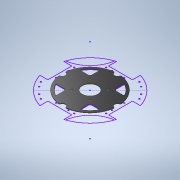
# Autodesk Inventor part: board
Saved by Autodesk Inventor 2020 (Build 240168000, 168)
## iProperties
Created: 2024-09-14
Part Number: board
Material: Типовые
Document SubType Name: Modeling
Designer: Ivan
Density: 1 g/cm^3
Appearance: Глянцевая — черная
Author: Ivan
Autodesk Inventor part; units mm, degrees
ref_plane "YZ Plane" through (0, 0, 0) normal (1, 0, 0) x (0, 1, 0)
ref_plane "XZ Plane" through (0, 0, 0) normal (0, 1, 0) x (-1, 0, 0)
ref_plane "XY Plane" through (0, 0, 0) normal (0, 0, 1) x (1, 0, 0)
sketch "Эскиз1" plane through (0, 0, 0) normal (0, 1, 0) x (-1, 0, 0)
  circle A0 centre (0, 0) radius 72.2724
  line L0 (46.8072, -8) -> (71.8282, -8)
  line L1 (46.8072, 8) -> (71.8282, 8)
  line L2 (-8, 46.8072) -> (-8, 71.8282)
  line L3 (8, 46.8072) -> (8, 71.8282)
  line L4 (-46.8072, -8) -> (-71.8282, -8)
  line L5 (-46.8072, 8) -> (-71.8282, 8)
  line L6 (8, -46.8072) -> (8, -71.8282)
  line L7 (-8, -46.8072) -> (-8, -71.8282)
  circle A1 centre (0, 0) radius 20
  point P0 (0, 0)
  point P1 (71.0292, -13.3471)
  point P2 (71.0292, 13.3471)
  constraints: 16 end point, 2 centre point, 1 horizontal, 1 point on circle
sketch "Эскиз4" plane through (0, 0, 0) normal (0, 1, 0) x (-1, 0, 0)
  line L0 (31, 34.7373) -> (31, 58.0259)
  line L1 (34.72, 31.0173) -> (58.0086, 31.0173)
  arc A0 (34.72, 31.0173) -> (31, 34.7373) centre (0, 0.0173) ccw
  arc A1 (58.0086, 31.0173) -> (31, 58.0259) centre (0, 0.0173) ccw
  line L2 (-58.0173, 31.0259) -> (-34.7286, 31.0259)
  arc A2 (-31.0086, 58.0346) -> (-58.0173, 31.0259) centre (-0.0086, 0.0259) ccw
  line L3 (-31.0086, 34.7459) -> (-31.0086, 58.0346)
  arc A3 (-31.0086, 34.7459) -> (-34.7286, 31.0259) centre (-0.0086, 0.0259) ccw
  line L4 (-31.0173, -57.9914) -> (-31.0173, -34.7027)
  arc A4 (-58.0259, -30.9827) -> (-31.0173, -57.9914) centre (-0.0173, 0.0173) ccw
  line L5 (-34.7373, -30.9827) -> (-58.0259, -30.9827)
  arc A5 (-34.7373, -30.9827) -> (-31.0173, -34.7027) centre (-0.0173, 0.0173) ccw
  line L6 (58, -30.9914) -> (34.7114, -30.9914)
  arc A6 (30.9914, -58) -> (58, -30.9914) centre (-0.0086, 0.0086) ccw
  line L7 (30.9914, -34.7114) -> (30.9914, -58)
  arc A7 (30.9914, -34.7114) -> (34.7114, -30.9914) centre (-0.0086, 0.0086) ccw
  point P0 (0, 0)
  point P1 (58, -31)
  dimension "d3" = 360
  constraints: 16 end point, 16 point on circle, 8 centre point, 3 coincident, 1 other
sketch "Эскиз2" plane through (0, 0, 0) normal (0, 1, 0) x (-1, 0, 0)
  circle A0 centre (0, 0) radius 72.2724 projected
  arc A1 (-8, 71.8282) -> (8, 71.8282) centre (0, 71.8282) ccw
  line L0 (31, 34.7373) -> (31, 58.0259) projected
  arc A2 (58.0086, 31.0173) -> (31, 58.0259) centre (0, 0.0173) ccw projected
  line L1 (34.72, 31.0173) -> (58.0086, 31.0173) projected
  arc A3 (34.72, 31.0173) -> (31, 34.7373) centre (0, 0.0173) ccw projected
  line L2 (31, 58.0259) -> (31, 34.7373)
  line L3 (34.72, 31.0173) -> (58.0086, 31.0173)
  arc A4 (34.72, 31.0173) -> (31, 34.7373) centre (0, 0.0173) ccw
  arc A5 (58.0086, 31.0173) -> (31, 58.0259) centre (0, 0.0173) ccw
  circle A6 centre (0, 0.0173) radius 56.1 construction
  line L4 (32.9126, 32.9299) -> (46.5081, 46.5254) construction
  line L5 (-58.0086, 31.0173) -> (-34.72, 31.0173)
  arc A7 (-31, 34.7373) -> (-34.72, 31.0173) centre (0, 0.0173) ccw
  line L6 (-31, 34.7373) -> (-31, 58.0259)
  arc A8 (-31, 58.0259) -> (-58.0086, 31.0173) centre (0, 0.0173) ccw
  line L7 (-31, -57.9914) -> (-31, -34.7027)
  arc A9 (-34.72, -30.9827) -> (-31, -34.7027) centre (0, 0.0173) ccw
  line L8 (-34.72, -30.9827) -> (-58.0086, -30.9827)
  arc A10 (-58.0086, -30.9827) -> (-31, -57.9914) centre (0, 0.0173) ccw
  line L9 (58.0086, -30.9827) -> (34.72, -30.9827)
  arc A11 (31, -34.7027) -> (34.72, -30.9827) centre (0, 0.0173) ccw
  line L10 (31, -34.7027) -> (31, -57.9914)
  arc A12 (31, -57.9914) -> (58.0086, -30.9827) centre (0, 0.0173) ccw
  arc A13 (-71.8282, -8) -> (-71.8282, 8) centre (-71.8282, 0) ccw
  arc A14 (8, -71.8282) -> (-8, -71.8282) centre (0, -71.8282) ccw
  arc A15 (71.8282, 8) -> (71.8282, -8) centre (71.8282, 0) ccw
  point P0 (0, 0)
  point P1 (-32.9126, 32.9299)
  point P2 (-46.5081, 46.5254)
  point P3 (-32.9126, -32.8953)
  point P4 (-46.5081, -46.4908)
  point P5 (32.9126, -32.8953)
  point P6 (46.5081, -46.4908)
  point P7 (58.0086, -30.9827)
  dimension "d0" = 8
  dimension "d4" = 112.2
  dimension "d7" = 360
  constraints: 26 point on circle, 18 end point, 13 centre point, 6 coincident, 3 equal radius, 2 collinear, 54 other
  measures "d0" radius of A1
  measures "d4" diameter of A6
extrude "Выдавливание1" add sketch "Эскиз2" along normal blind 1.3 contours A15 A0 A14 A13 A1
fillet "Сопряжение1" radius 2 24 edges at (-58.0086, 0.65, 31.0173) (-34.72, 0.65, 31.0173) (-31, 0.65, 34.7373) (-31, 0.65, 58.0259) (-8, 0.65, 71.8282) (8, 0.65, 71.8282) (58.0086, 0.65, 31.0173) (34.72, 0.65, 31.0173) (31, 0.65, 34.7373) (31, 0.65, 58.0259) (71.8282, 0.65, -8) (71.8282, 0.65, 8) (31, 0.65, -34.7027) (34.72, 0.65, -30.9827) (-8, 0.65, -71.8282) (8, 0.65, -71.8282) (31, 0.65, -57.9914) (58.0086, 0.65, -30.9827) (-31, 0.65, -34.7027) (-34.72, 0.65, -30.9827) (-31, 0.65, -57.9914) (-58.0086, 0.65, -30.9827) (-71.8282, 0.65, -8) (-71.8282, 0.65, 8)
sketch "Эскиз5" plane through (0, 1.3, 0) normal (0, 1, 0) x (1, 0, 0)
  circle A0 centre (0, 0) radius 20
  circle A1 centre (0, 0) radius 33.25 construction
  line L0 (0, 0) -> (23.5113, 23.5113) construction
  line L1 (0, 0) -> (33.25, 0) construction
  circle A2 centre (23.5113, 23.5113) radius 2.15
  circle A3 centre (-23.5113, 23.5113) radius 2.15
  circle A4 centre (-23.5113, -23.5113) radius 2.15
  circle A5 centre (23.5113, -23.5113) radius 2.15
  dimension "d16" = 66.5
  dimension "d13" = 40
  dimension "d17" = 45
  dimension "d18" = 4.3
  dimension "d21" = 360
  constraints: 5 centre point, 4 end point, 3 coincident, 1 equal length, 1 horizontal, 12 other
  measures "d13" diameter of A0
  measures "d17" angle of L1 L0
  measures "d18" diameter of A2
extrude "Выдавливание2" cut sketch "Эскиз5" against normal blind 1.3
sketch "Эскиз6" plane through (0, 0, 0) normal (0, -1, 0) x (1, 0, 0)
  arc A0 (-31, 99.2724) -> (-99.2724, 31) centre (0, 0) ccw
  circle A1 centre (-74.5664, 57.67) radius 1.5
  circle A2 centre (-82.9015, 44.87) radius 1.5
  circle A3 centre (-57.67, 74.5664) radius 1.5
  circle A4 centre (-44.87, 82.9015) radius 1.5
  line L0 (-31, 99.2724) -> (-31, 78.7724)
  line L1 (-31, 78.7724) -> (31, 78.7724)
  circle A5 centre (-16, 72.43) radius 1.5
  circle A6 centre (16, 72.43) radius 1.5
  circle A7 centre (31, 72.43) radius 1.5
  line L2 (31, 78.7724) -> (31, 99.2724)
  circle A8 centre (16, 42.22) radius 1.5
  circle A9 centre (-16, 42.22) radius 1.5
  circle A10 centre (-42.22, 16) radius 1.5
  circle A11 centre (-72.43, 16) radius 1.5
  line L3 (-99.2724, 31) -> (-78.7724, 31)
  line L4 (-78.7724, 31) -> (-78.7724, -31)
  arc A12 (34.57, 98.0863) -> (98.0863, 34.57) centre (109.0212, 109.0212) ccw
  circle A13 centre (72.43, 31) radius 1.5
  line L5 (99.2724, 31) -> (78.7724, 31)
  line L6 (78.7724, 31) -> (78.7724, -31)
  circle A14 centre (72.43, 16) radius 1.5
  circle A15 centre (42.22, 16) radius 1.5
  circle A16 centre (42.22, -16) radius 1.5
  circle A17 centre (72.43, -16) radius 1.5
  circle A18 centre (82.9015, -44.87) radius 1.5
  line L7 (78.7724, -31) -> (99.2724, -31)
  arc A19 (31, -99.2724) -> (99.2724, -31) centre (0, 0) ccw
  circle A20 centre (74.5664, -57.67) radius 1.5
  circle A21 centre (16, -42.22) radius 1.5
  circle A22 centre (57.67, -74.5664) radius 1.5
  circle A23 centre (44.87, -82.9015) radius 1.5
  circle A24 centre (16, -72.43) radius 1.5
  line L8 (31, -78.7724) -> (31, -99.2724)
  line L9 (-31, -78.7724) -> (31, -78.7724)
  circle A25 centre (-16, -72.43) radius 1.5
  circle A26 centre (-16, -42.22) radius 1.5
  circle A27 centre (-31, -72.43) radius 1.5
  circle A28 centre (-42.22, -16) radius 1.5
  circle A29 centre (-72.43, -16) radius 1.5
  circle A30 centre (-72.43, -31) radius 1.5
  line L10 (-78.7724, -31) -> (-99.2724, -31)
  line L11 (-31, -99.2724) -> (-31, -78.7724)
  arc A31 (-34.57, -98.0863) -> (-31, -99.2724) centre (0, 0) ccw
  arc A32 (-99.2724, -31) -> (-98.0863, -34.57) centre (0, 0) ccw
  arc A33 (-34.57, -98.0863) -> (-98.0863, -34.57) centre (-109.0212, -109.0212) ccw
  line L12 (-73.5391, 73.5391) -> (73.5391, -73.5391) construction
  arc A34 (34.57, 98.0863) -> (31, 99.2724) centre (0, 0) ccw
  arc A35 (99.2724, 31) -> (98.0863, 34.57) centre (0, 0) ccw
  arc A36 (-98.0863, -34.57) -> (-34.57, -98.0863) centre (0, 0) ccw
  arc A37 (98.0863, 34.57) -> (34.57, 98.0863) centre (0, 0) ccw
  constraints: 38 centre point, 26 end point, 23 point on circle, 5 coincident, 1 horizontal, 1 perpendicular, 1 symmetric about line, 2 other
